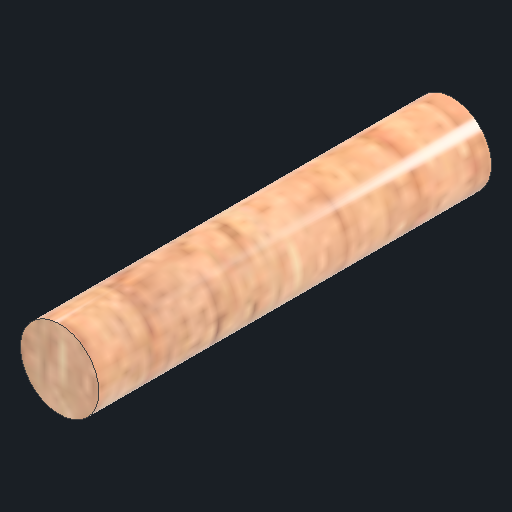
# Autodesk Inventor part: MAIN_PIVOT_DOWEL_TREBUCHET
Saved by Autodesk Inventor 2026.2 (Build 302298010, 298A)
## iProperties
Created: 2026-02-19
Part Number: MAIN_PIVOT_DOWEL_TREBUCHET
Material: Wood (Birch)
Document SubType Name: Modeling
Designer: 4aida
Density: 0.55 g/cm^3
Appearance: Birch - Natural Polished
Mass: 4.42419 g
Surface Area: 27.8689 cm^2
Volume: 8.04398 cm^3
Author: 4aida
Autodesk Inventor part; units mm, degrees
ref_plane "YZ Plane" through (0, 0, 0) normal (1, 0, 0) x (0, 1, 0)
ref_plane "XZ Plane" through (0, 0, 0) normal (0, 1, 0) x (-1, 0, 0)
ref_plane "XY Plane" through (0, 0, 0) normal (0, 0, 1) x (1, 0, 0)
sketch "Sketch1" plane through (0, 0, 0) normal (0, 0, 1) x (1, 0, 0)
  circle A0 centre (0, 0) radius 6.35
  dimension "d0" = 12.7
  constraints: 1 centre point, 1 coincident
  measures "d0" diameter of A0
extrude "Extrusion1" add sketch "Sketch1" along normal mid plane 63.5
body "Solid1"
